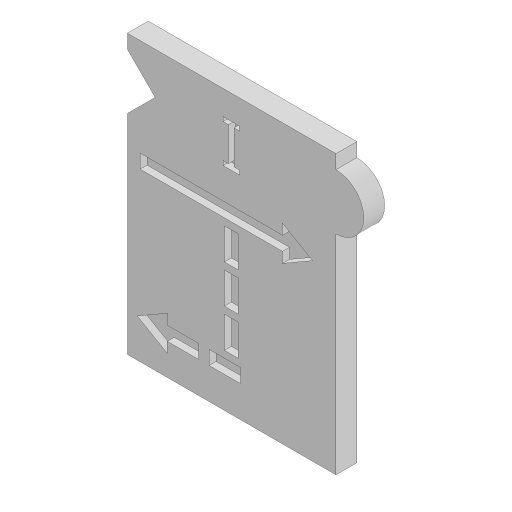
# Autodesk Inventor part: MS_I[203] text
Saved by Autodesk Inventor 2023 (Build 270158000, 158)
## iProperties
Created: 2023-03-29
Part Number: MS_I[203] text
Material: Generic
Document SubType Name: Modeling
Designer: LKLM8608
Density: 1 g/cm^3
Appearance: Default
Author: LKLM8608
Autodesk Inventor part; units mm, degrees
ref_plane "YZ Plane" through (0, 0, 0) normal (1, 0, 0) x (0, 1, 0)
ref_plane "XZ Plane" through (0, 0, 0) normal (0, 1, 0) x (-1, 0, 0)
ref_plane "XY Plane" through (0, 0, 0) normal (0, 0, 1) x (1, 0, 0)
sketch "Sketch1" plane through (0, 0, 0) normal (0, 0, 1) x (1, 0, 0)
  line L0 (0, 0) -> (-30, 0)
  line L1 (-30, 40) -> (0, 40)
  line L2 (-36.1318, 34) -> (13.8682, 34) construction
  arc A0 (0, 30) -> (0, 38) centre (0, 34) ccw
  circle A1 centre (-30, 34) radius 4 construction
  line L3 (-30, 30) -> (0, 30) construction
  line L4 (-30, 38) -> (-26, 34)
  line L5 (-30, 30) -> (-26, 34)
  line L6 (0, 40) -> (0, 38)
  line L7 (0, 30) -> (0, 0)
  line L8 (-30, 0) -> (-30, 30)
  line L9 (-30, 38) -> (-30, 40)
  dimension "d0" = 30
  dimension "d1" = 40
  dimension "d3" = 6
  dimension "d4" = 8
  dimension "d5" = 8
  dimension "d6" = 30
  constraints: 20 end point, 5 parallel, 5 point on circle, 3 perpendicular, 3 point on line, 2 centre point, 2 horizontal
  measures "d0" distance of L1.start L1.end
  measures "d1" distance of L0.end L1.start
  measures "d3" distance between parallel lines of L2 L1
  measures "d4" diameter of A0
  measures "d5" diameter of A1
  measures "d6" distance between parallel lines of L0 L3
extrude "Extrusion1" add sketch "Sketch1" along normal blind 3
sketch "Sketch3" plane through (0, 0, 3) normal (0, 0, 1) x (1, 0, 0)
  line L0 (-30, 40) -> (0, 40) construction
  line L1 (-30, 0) -> (-30, 30) construction
  line L2 (0, 0) -> (-30, 0) construction
  line L3 (-15.0586, 25.9999) -> (-30, 25.9849) construction
  line L4 (-28.1581, 25.9868) -> (-7.691, 25.9868)
  line L5 (-7.691, 25.9868) -> (-7.691, 23.9868)
  line L6 (-28.1581, 23.9868) -> (-28.1581, 25.9868)
  line L7 (-7.691, 24.9868) -> (-1.5179, 24.9868) construction
  line L8 (-7.691, 25.9868) -> (-7.691, 27.4868)
  line L9 (-7.691, 27.4868) -> (-3.3609, 24.9868)
  line L10 (-7.691, 23.9868) -> (-7.691, 22.4868)
  line L11 (-7.691, 22.4868) -> (-3.3609, 24.9868)
  line L12 (-14.0467, 18.4868) -> (-16.0467, 18.4868)
  line L13 (-16.0467, 18.4868) -> (-16.0467, 22.9868)
  line L14 (-16.0467, 22.9868) -> (-14.0467, 22.9868)
  line L15 (-14.0467, 22.9868) -> (-14.0467, 18.4868)
  line L16 (-14.0467, 18.4868) -> (-16.0467, 22.9868) construction
  line L17 (-16.0467, 18.4868) -> (-14.0467, 22.9868) construction
  line L18 (-15, 0) -> (-15.0135, 6) construction
  line L19 (-15.0135, 6) -> (-28.7905, 6) construction
  line L20 (-13.75, 6.5) -> (-18.25, 6.5)
  line L21 (-18.25, 6.5) -> (-18.25, 4.5)
  line L22 (-18.25, 4.5) -> (-13.75, 4.5)
  line L23 (-13.75, 4.5) -> (-13.75, 6.5)
  line L24 (-19.75, 6.5) -> (-24.25, 6.5)
  line L25 (-19.75, 4.5) -> (-19.75, 6.5)
  line L26 (-24.25, 4.5) -> (-19.75, 4.5)
  line L27 (-24.25, 6.5) -> (-24.25, 4.5)
  line L28 (-24.25, 5.5) -> (-29.2128, 5.5) construction
  line L29 (-24.25, 6.5) -> (-24.25, 8)
  line L30 (-24.25, 8) -> (-28.5801, 5.5)
  line L31 (-24.25, 4.5) -> (-24.25, 3)
  line L32 (-24.25, 3) -> (-28.5801, 5.5)
  line L33 (-16.616, 36.5) -> (-11.3751, 36.5) construction
  line L34 (-11.3751, 36.5) -> (-11.3751, 28.9531) construction
  line L35 (-11.3751, 28.9531) -> (-16.616, 28.9531) construction
  line L36 (-16.616, 28.9531) -> (-16.616, 36.5) construction
  line L37 (-16.25, 40) -> (-16.25, 36.4806) construction
  line L38 (-28.1581, 23.9868) -> (-7.691, 23.9868)
  line L39 (-16.0467, 17.4868) -> (-14.0467, 17.4868)
  line L40 (-14.0467, 17.4868) -> (-14.0467, 12.9868)
  line L41 (-16.0467, 12.9868) -> (-16.0467, 17.4868)
  line L42 (-14.0467, 12.9868) -> (-16.0467, 12.9868)
  line L43 (-16.0467, 12.9868) -> (-14.0467, 17.4868) construction
  line L44 (-14.0467, 12.9868) -> (-16.0467, 17.4868) construction
  line L45 (-16.0467, 11.9868) -> (-14.0467, 11.9868)
  line L46 (-14.0467, 11.9868) -> (-14.0467, 7.4868)
  line L47 (-16.0467, 7.4868) -> (-16.0467, 11.9868)
  line L48 (-14.0467, 7.4868) -> (-16.0467, 7.4868)
  line L49 (-16.0467, 7.4868) -> (-14.0467, 11.9868) construction
  line L50 (-14.0467, 7.4868) -> (-16.0467, 11.9868) construction
  line L51 (-13.8725, 30.4) -> (-16.2354, 30.4)
  line L52 (-16.2354, 30.4) -> (-16.2354, 31.0229)
  line L53 (-16.2354, 31.0229) -> (-15.4593, 31.0229)
  line L54 (-15.4593, 31.0229) -> (-15.4593, 35.8771)
  line L55 (-15.4593, 35.8771) -> (-16.2354, 35.8771)
  line L56 (-16.2354, 35.8771) -> (-16.2354, 36.5)
  line L57 (-16.2354, 36.5) -> (-13.8725, 36.5)
  line L58 (-13.8725, 36.5) -> (-13.8725, 35.8771)
  line L59 (-13.8725, 35.8771) -> (-14.6486, 35.8771)
  line L60 (-14.6486, 35.8771) -> (-14.6486, 31.0229)
  line L61 (-14.6486, 31.0229) -> (-13.8725, 31.0229)
  line L62 (-13.8725, 31.0229) -> (-13.8725, 30.4)
  point P0 (-15.0467, 20.7368)
  point P1 (-15.0467, 15.2368)
  point P2 (-15.0467, 9.7368)
  point P3 (-15, 40)
  point P4 (-15, 40)
  dimension "d10" = 26
  dimension "d11" = 2
  dimension "d12" = 1.5
  dimension "d13" = 5
  dimension "d14" = 1.5
  dimension "d15" = 2
  dimension "d16" = 4.5
  dimension "d24" = 6
  dimension "d25" = 4.5
  dimension "d26" = 2
  dimension "d29" = 6
  dimension "d34" = 1.5
  dimension "d35" = 5
  dimension "d36" = 1.5
  dimension "d39" = 8
  dimension "d40" = 1
  dimension "d48" = 5.5
  dimension "d53" = 3.5
  dimension "d54" = 14
  constraints: 88 end point, 7 horizontal, 7 midpoint, 5 parallel, 5 point on line, 5 vertical, 4 perpendicular, 1 collinear, 31 other
  measures "d10" distance of L18.start L3.start
  measures "d11" distance of L4.end L5.end
  measures "d12" distance of L4.end L8.end
  measures "d13" distance of L8.end L9.end
  measures "d14" distance of L5.end L10.end
  measures "d15" distance of L13.end L14.end
  measures "d16" distance of L12.end L13.end
  measures "d24" distance of L18.start L18.end
  measures "d25" distance of L22.end L21.end
  measures "d26" distance of L21.end L20.end
  measures "d29" distance of L20.start L24.start
  measures "d34" distance of L24.end L29.end
  measures "d35" distance of L29.end L30.end
  measures "d36" distance of L26.start L31.end
  measures "d39" distance from line of L2 L29.end
  measures "d40" distance between parallel lines of L38 L14
  measures "d48" distance of L13.end L39.start
  measures "d53" distance from line of point (-15, 40) L33
  measures "d54" distance from line of point (-15, 40) L3
extrude "Extrusion2" cut sketch "Sketch3" against normal blind 1
body "Solid1"
